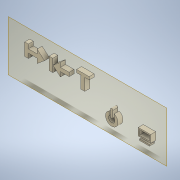
# Autodesk Inventor part: InterfacePlateTextOrange
Saved by Autodesk Inventor 2022 (Build 260153000, 153)
## iProperties
Created: 2022-02-05
Part Number: InterfacePlateTextOrange
Material: Generic
Document SubType Name: Modeling
Designer: siwat
Density: 1 g/cm^3
Appearance: Default
VLDS_Profile: Default Part
VLDS_TimeStamp: 2022-02-27
VLDS_FailCnt: 0
VLDS_AcceptCnt: 0
Author: siwat
Autodesk Inventor part; units mm, degrees
ref_plane "YZ Plane" through (0, 0, 0) normal (1, 0, 0) x (0, 1, 0)
ref_plane "XZ Plane" through (0, 0, 0) normal (0, 1, 0) x (-1, 0, 0)
ref_plane "XY Plane" through (0, 0, 0) normal (0, 0, 1) x (1, 0, 0)
ref_plane "Work Plane1" through (0, 0, 0) normal (0, 0, 1) x (1, 0, 0)
sketch "Sketch1" plane through (0, 0, 0) normal (0, 0, 1) x (1, 0, 0)
  line L0 (-25.2022, 4.5916) -> (-23.7022, 4.5916)
  line L1 (-23.7022, 4.5916) -> (-23.7022, -0.4084)
  line L2 (-23.7022, -0.4084) -> (-25.2022, -0.4084)
  line L3 (-25.2022, -0.4084) -> (-25.2022, 4.5916)
  line L4 (-23.7022, 2.9563) -> (-20.2022, 2.9563)
  line L5 (-20.2022, 2.9563) -> (-20.2022, 1.4563)
  line L6 (-20.2022, 1.4563) -> (-23.7022, 1.4563)
  line L7 (-20.2022, 2.9563) -> (-20.2022, 4.5916)
  line L8 (-20.2022, 4.5916) -> (-17.2022, 2.0916)
  line L9 (-17.2022, 2.0916) -> (-20.2022, -0.4084)
  line L10 (-20.2022, -0.4084) -> (-20.2022, 1.4563)
  line L11 (-4.3885, 5.4681) -> (0.6682, 5.4681) construction
  line L12 (0.6682, 5.4681) -> (0.6682, -0.5319) construction
  line L13 (0.6682, -0.5319) -> (-4.3885, -0.5319) construction
  line L14 (-4.3885, -0.5319) -> (-4.3885, 5.4681) construction
  line L15 (-15.3667, 4.5916) -> (-13.8667, 4.5916)
  line L16 (-13.8667, 4.5916) -> (-13.8667, -0.4084)
  line L17 (-13.8667, -0.4084) -> (-15.3667, -0.4084)
  line L18 (-15.3667, -0.4084) -> (-15.3667, 4.5916)
  line L19 (-13.8667, 2.2063) -> (-10.8667, 4.5916)
  line L20 (-13.8667, 2.2063) -> (-10.8667, -0.4084)
  line L21 (-10.8667, 4.5916) -> (-10.8667, -0.4084)
  line L22 (-10.8667, 2.9563) -> (-7.3667, 2.9563)
  line L23 (-7.3667, 2.9563) -> (-7.3667, 1.4563)
  line L24 (-7.3667, 1.4563) -> (-10.8667, 1.4563)
  line L25 (-10.8667, 1.4563) -> (-10.8667, 2.9563)
  circle A0 centre (9.7092, -4.736) radius 2.5
  circle A1 centre (9.7092, -4.736) radius 1.25
  line L26 (9.7092, -0.9774) -> (9.7092, -0.9774)
  line L27 (10.2092, -1.4774) -> (10.2092, -3.9774)
  line L28 (9.7092, -4.4774) -> (9.7092, -4.4774)
  line L29 (9.2092, -3.9774) -> (9.2092, -1.4774)
  arc A2 (9.7092, -4.4774) -> (10.2092, -3.9774) centre (9.7092, -3.9774) ccw
  arc A3 (9.2092, -3.9774) -> (9.7092, -4.4774) centre (9.7092, -3.9774) ccw
  arc A4 (9.7092, -0.9774) -> (9.2092, -1.4774) centre (9.7092, -1.4774) ccw
  arc A5 (10.2092, -1.4774) -> (9.7092, -0.9774) centre (9.7092, -1.4774) ccw
  line L30 (8.7092, -2.4447) -> (8.7092, -3.986)
  line L31 (10.7092, -2.4447) -> (10.7092, -3.986)
  line L32 (20.3303, -2.3036) -> (25.3303, -2.3036)
  line L33 (25.3303, -2.3036) -> (25.3303, -5.3036)
  line L34 (25.3303, -5.3036) -> (20.3303, -5.3036)
  line L35 (20.3303, -5.3036) -> (20.3303, -2.3036)
  line L36 (20.8303, -2.8036) -> (24.8303, -2.8036)
  line L37 (24.8303, -2.8036) -> (24.8303, -4.8036)
  line L38 (24.8303, -4.8036) -> (20.8303, -4.8036)
  line L39 (20.8303, -4.8036) -> (20.8303, -2.8036)
  line L40 (20.8303, -6.0266) -> (24.8303, -6.0266)
  line L41 (24.8303, -6.0266) -> (24.8303, -6.5869)
  line L42 (24.8303, -6.5869) -> (20.8303, -6.5869)
  line L43 (20.8303, -6.5869) -> (20.8303, -6.0266)
  line L44 (-2.6138, -0.5319) -> (-2.6138, 4.3255)
  line L45 (-2.6138, 4.3255) -> (-4.3885, 4.3255)
  line L46 (-4.3885, 4.3255) -> (-4.3885, 5.4681)
  line L47 (-4.3885, 5.4681) -> (0.6682, 5.4681)
  line L48 (0.6682, 5.4681) -> (0.6682, 4.3255)
  line L49 (0.6682, 4.3255) -> (-1.1065, 4.3255)
  line L50 (-1.1065, 4.3255) -> (-1.1065, -0.5319)
  line L51 (-1.1065, -0.5319) -> (-2.6138, -0.5319)
  point P0 (0, 0)
  point P1 (10.2092, -4.4774)
  point P2 (10.2092, -0.9774)
  point P3 (9.2092, -4.4774)
  point P4 (20.8303, -3.8036)
  dimension "d0" = 1.5
  dimension "d1" = 5
  dimension "d2" = 1.5
  dimension "d3" = 3.5
  dimension "d4" = 3
  dimension "d5" = 1.5
  dimension "d6" = 5
  dimension "d7" = 3
  dimension "d8" = 3.5
  dimension "d9" = 1.5
  dimension "d10" = 5
  dimension "d11" = 2.5
  dimension "d12" = 1
  dimension "d13" = 3.5
  dimension "d14" = 0.5
  dimension "d15" = 0.5
  dimension "d16" = 0.5
  dimension "d17" = 0.5
  dimension "d20" = 5
  dimension "d21" = 3
  dimension "d22" = 4
  dimension "d23" = 2
  dimension "d24" = 0.5
  dimension "d25" = 0.5
  constraints: 80 end point, 15 parallel, 12 point on circle, 11 point on line, 9 perpendicular, 8 horizontal, 8 tangent, 6 centre point, 3 equal radius, 3 vertical, 1 coincident, 1 collinear, 1 midpoint, 2 other
  measures "d0" distance of L1.end L2.end
  measures "d1" distance of L0.end L1.end
  measures "d2" distance of L4.end L5.end
  measures "d3" distance of L4.start L4.end
  measures "d4" distance from line of L5 L8.end
  measures "d5" distance of L16.end L17.end
  measures "d6" distance of L15.end L16.end
  measures "d7" distance between parallel lines of L16 L21
  measures "d8" distance of L23.end L24.end
  measures "d9" distance of L22.end L23.end
  measures "d10" diameter of A0
  measures "d11" diameter of A1
  measures "d12" distance of point (10.209, -4.477) point (9.209, -4.477)
  measures "d13" distance of point (10.209, -0.977) point (10.209, -4.477)
  measures "d14" distance from line of L27 A0.centre
  measures "d15" radius of A2
  measures "d16" distance between parallel lines of L31 L27
  measures "d17" distance between parallel lines of L30 L29
  measures "d20" distance of L33.end L34.end
  measures "d21" distance of L32.end L33.end
  measures "d22" distance of L37.end L38.end
  measures "d23" distance of L36.end L37.end
  measures "d24" distance between parallel lines of L36 L32
  measures "d25" distance from line of L35 point (20.83, -3.804)
extrude "Extrusion1" add sketch "Sketch1" against normal blind 2 contours L0 L1 L2 L3 | L4 L5 L6 L1 | L7 L8 L9 L10 L5 | L19 L21 L20 | L15 L16 L17 L18 | L22 L23 L24 L21 | A0 L30 A1 L31 | L27 A1 L29 A0 | A0 L29 A4 A5 L27 | L27 A2 A3 L29 A1 | L32 L33 L34 L35 | L40 L41 L42 L43 | L44 L45 L46 L47 L48 L49 L50 L51 picked at (9.961, -3.6586)
body "Solid1"
